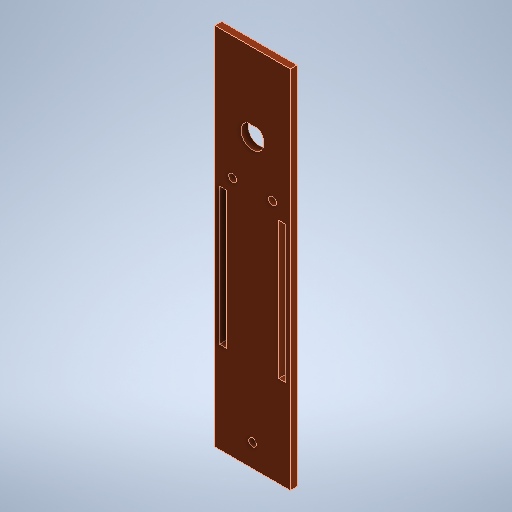
# Autodesk Inventor part: Motor Fixation .1
Saved by Autodesk Inventor 2025.4 (Build 294407000, 407)
## iProperties
Created: 2026-04-06
Part Number: Motor Fixation .1
Material: Generic
Document SubType Name: Sheet Metal
Designer: lenovo
Density: 1 g/cm^3
Sheet Metal Rule: Default_mm
Appearance: Default(1)
Author: lenovo
Autodesk Inventor part; units mm, degrees
ref_plane "YZ Plane" through (0, 0, 0) normal (1, 0, 0) x (0, 1, 0)
ref_plane "XZ Plane" through (0, 0, 0) normal (0, 1, 0) x (-1, 0, 0)
ref_plane "XY Plane" through (0, 0, 0) normal (0, 0, 1) x (1, 0, 0)
sketch "Sketch1" plane through (0, 0, 0) normal (0, 0, 1) x (1, 0, 0)
  line L0 (-16.5, -70) -> (16.5, -70)
  line L1 (16.5, -70) -> (16.5, 70)
  line L2 (16.5, 70) -> (-16.5, 70)
  line L3 (-16.5, 70) -> (-16.5, -70)
  line L4 (-16.5, -70) -> (16.5, 70) construction
  line L5 (16.5, -70) -> (-16.5, 70) construction
  line L6 (0, 70) -> (0, -70)
  line L7 (11.5, 30) -> (14.5, 30)
  line L8 (14.5, 30) -> (14.5, -30)
  line L9 (14.5, -30) -> (11.5, -30)
  line L10 (11.5, -30) -> (11.5, 30)
  circle A0 centre (0, 56) radius 5
  line L11 (-11.5, 30) -> (-14.5, 30)
  line L12 (-14.5, 30) -> (-14.5, -30)
  line L13 (-14.5, -30) -> (-11.5, -30)
  line L14 (-11.5, -30) -> (-11.5, 30)
  circle A1 centre (0, -60) radius 1.7
  circle A2 centre (-8.75, 36) radius 1.7
  circle A3 centre (8.75, 36) radius 1.7
  line L15 (-2.7129, 60.2) -> (2.7129, 60.2)
  point P0 (0, 0)
  point P1 (14.5, 0)
  point P2 (16.5, 0)
  point P3 (-14.5, 0)
  dimension "d1" = 140
  dimension "d2" = 3
  dimension "d3" = 2
  dimension "d4" = 60
  dimension "d5" = 10
  dimension "d6" = 14
  dimension "d7" = 3.4
  dimension "d8" = 10
  dimension "d9" = 3.4
  dimension "d10" = 23
  dimension "d11" = 20
  dimension "d21" = 4.2
  dimension "d22" = 17.5
  measures "d1" distance of L0.end L1.end
  measures "d2" distance of L7.start L7.end
  measures "d3" distance between parallel lines of L1 L8
  measures "d4" distance of L7.end L8.end
  measures "d5" diameter of A0
  measures "d6" distance from line of L2 A0.centre
  measures "d7" diameter of A1
  measures "d8" distance from line of L0 A1.centre
  measures "d9" diameter of A2
  measures "d10" distance between parallel lines of L10 L14
  measures "d11" vertical distance of A0.centre A2.centre
  measures "d21" distance from line of L15 A0.centre
  measures "d22" diameter of A2.centre L6
sketch "Sketch3" plane through (0, 0, 1.5) normal (0, 0, 1) x (1, 0, 0)
  line L0 (-16.5, 70) -> (-16.5, -70)
  line L1 (-16.5, 70) -> (16.5, 70)
  line L2 (16.5, 70) -> (16.5, 90)
  line L3 (16.5, 90) -> (-16.5, 90)
  line L4 (-16.5, 90) -> (-16.5, 70)
  line L5 (16.5, 70) -> (16.5, -70)
  point P0 (0, 0)
  point P1 (16.5, 0)
  dimension "d24" = 20
  measures "d24" distance of L1.end L2.end
extrude "Plate1" add sketch "Sketch1" along normal mid plane 3 contours L3 L2 L6 A0 A1 L0 | L6 A1 A0 L2 L1 L0 | A0 L15 L6 | L6 L15 A0 picked at (1.5261, 60.3463) picked at (-1.5261, 60.3463)
sheet face with bend "Face3" sketch "Sketch3" thickness 3 toward (0, 0, -1) bend radius 3
bend "Bend2"
equation "\"d13\" = Thickness"
equation "\"d25\" = BendRadius"
equation "\"d26\" = BendReliefWidth"
equation "\"d28\" = MinimumRemnant"
equation "\"d27\" = BendReliefDepth"
equation "\"d29\" = TransitionRadius"
equation "\"BendRadius\" = Thickness"
equation "\"BendReliefWidth\" = Thickness"
equation "\"BendReliefDepth\" = 0.5 * Thickness"
equation "\"CornerReliefSize\" = 4 * Thickness"
equation "\"MinimumRemnant\" = 2 * Thickness"
equation "\"TransitionRadius\" = BendRadius"
equation "\"JacobiRadiusSize\" = BendRadius"
equation "\"GapSize\" = Thickness"
equation "\"Thickness\" = 3"
body "Solid1"
